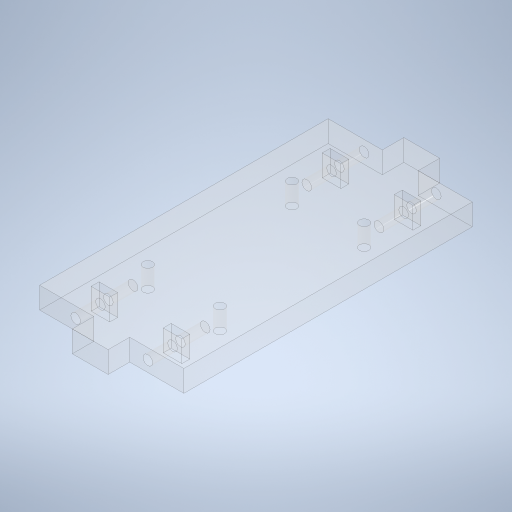
# Autodesk Inventor part: feet_holder3
Saved by Autodesk Inventor 2024 (Build 280153000, 153)
## iProperties
Created: 2024-09-07
Part Number: feet_holder3
Material: PMMA 플라스틱
Document SubType Name: Modeling
Designer: jmha0
Density: 1.188 g/cm^3
Appearance: 폴리카보네이트 - 선명
Mass: 23.3204 g
Surface Area: 87.9044 cm^2
Volume: 19.63 cm^3
Author: jmha0
Autodesk Inventor part; units mm, degrees
ref_plane "YZ Plane" through (0, 0, 0) normal (1, 0, 0) x (0, 1, 0)
ref_plane "XZ Plane" through (0, 0, 0) normal (0, 1, 0) x (-1, 0, 0)
ref_plane "XY Plane" through (0, 0, 0) normal (0, 0, 1) x (1, 0, 0)
sketch "스케치1" plane through (0, 0, 0) normal (0, 1, 0) x (-1, 0, 0)
  circle A0 centre (7.6948, -23.9851) radius 1.45
  circle A1 centre (27.7948, -23.9851) radius 1.45
  line L0 (-2.3552, -20.9851) -> (37.8448, -20.9851)
  line L1 (-2.3552, -20.9851) -> (-2.3552, -26.9851)
  line L2 (37.8448, -26.9851) -> (-2.3552, -26.9851)
  line L3 (37.8448, -20.9851) -> (37.8448, -26.9851)
  circle A2 centre (27.7948, 62.4149) radius 1.45
  circle A3 centre (7.6948, 62.4149) radius 1.45
  line L4 (37.8448, 65.4149) -> (-2.3552, 65.4149)
  line L5 (-2.3552, 65.4149) -> (-2.3552, 59.4149)
  line L6 (37.8448, 59.4149) -> (-2.3552, 59.4149)
  line L7 (37.8448, 65.4149) -> (37.8448, 59.4149)
  line L8 (37.8448, -20.9851) -> (-2.3552, -20.9851)
  line L9 (-2.3552, -20.9851) -> (-2.3552, 59.4149)
  line L10 (-2.3552, 59.4149) -> (37.8448, 59.4149)
  line L11 (37.8448, 59.4149) -> (37.8448, -20.9851)
  point P0 (0, 0)
  constraints: 24 end point, 4 centre point, 2 parallel, 1 horizontal, 1 perpendicular
extrude "돌출1" add sketch "스케치1" along normal blind 6 contours L9 L6 L11 L0
sketch "스케치2" plane through (0, 6, 0) normal (0, 1, 0) x (1, 0, 0)
  line L0 (2.3552, 20.9851) -> (-37.8448, 20.9851) projected
  line L1 (-37.8448, 20.9851) -> (-37.8448, -59.4149) projected
  line L2 (-37.8448, -59.4149) -> (2.3552, -59.4149) projected
  line L3 (2.3552, -59.4149) -> (2.3552, 20.9851) projected
  line L4 (-47.7448, 30.7851) -> (12.2552, -69.2149) construction
  line L5 (12.2552, 30.7851) -> (-47.7448, -69.2149) construction
  circle A0 centre (-7.6948, -39.3149) radius 1.35
  circle A1 centre (-27.7948, -39.3149) radius 1.35
  circle A2 centre (-7.6948, 0.8851) radius 1.35
  circle A3 centre (-27.7948, 0.8851) radius 1.35
  point P0 (0, 0)
  dimension "d2" = 60
  dimension "d3" = 100
  dimension "d4" = 2.7
  dimension "d5" = 2.7
  dimension "d6" = 2.7
  dimension "d27" = 2.7
  constraints: 4 centre point, 4 end point
  measures "d2" distance of L4.end L5.end
  measures "d3" distance of L5.start L4.end
  measures "d4" diameter of A0
  measures "d5" diameter of A2
  measures "d6" diameter of A3
  measures "d27" diameter of A1
extrude "돌출2" cut sketch "스케치2" against normal blind 6 contours A0 | A1 | A2 | A3
sketch "스케치3" plane through (-37.8448, 0, 59.4149) normal (0, 0, 1) x (1, 0, 0)
  line L0 (0, 0) -> (40.2, 0) projected
  line L1 (40.2, 0) -> (40.2, 6) projected
  line L2 (0, 6) -> (40.2, 6) projected
  line L3 (0, 0) -> (0, 6) projected
  line L4 (0, 6) -> (10.05, 6)
  line L5 (10.05, 6) -> (30.15, 6)
  circle A0 centre (10.05, 3) radius 1.35
  circle A1 centre (30.15, 3) radius 1.35
  point P0 (37.8448, 0)
  dimension "d9" = 40.2
  dimension "d10" = 6
  dimension "d11" = 10.05
  dimension "d12" = 20.1
  dimension "d13" = 2.7
  dimension "d14" = 2.7
  constraints: 4 end point, 2 centre point, 2 point on line
  measures "d9" distance of L2.start L1.end
  measures "d10" distance of L0.start L2.start
  measures "d11" distance of L2.start L4.end
  measures "d12" distance of L4.end L5.end
  measures "d13" diameter of A0
  measures "d14" diameter of A1
extrude "돌출3" cut sketch "스케치3" against normal blind 16 contours A0 | A1
sketch "스케치4" plane through (2.3552, 0, -20.9851) normal (0, 0, -1) x (-1, 0, 0)
  circle A0 centre (30.15, 3) radius 1.35 projected
  line L0 (11.4, 6) -> (11.4, 0) projected
  circle A1 centre (10.05, 3) radius 1.35 projected
  point P0 (2.3552, 0)
extrude "돌출4" cut sketch "스케치4" against normal blind 16
sketch "스케치5" plane through (0, 6, 0) normal (0, 1, 0) x (1, 0, 0)
  line L0 (-29.1448, 20.9851) -> (-29.1448, 4.9851) projected
  line L1 (-26.4448, 20.9851) -> (-26.4448, 4.9851) projected
  line L2 (-29.1448, 4.9851) -> (-26.4448, 4.9851) projected
  line L3 (-9.0448, 20.9851) -> (-9.0448, 4.9851) projected
  line L4 (-6.3448, 20.9851) -> (-6.3448, 4.9851) projected
  line L5 (-9.0448, 4.9851) -> (-6.3448, 4.9851) projected
  circle A0 centre (-7.6948, 0.8851) radius 1.35 projected
  circle A1 centre (-27.7948, 0.8851) radius 1.35 projected
  circle A2 centre (-7.6948, -39.3149) radius 1.35 projected
  circle A3 centre (-27.7948, -39.3149) radius 1.35 projected
  line L6 (2.3552, 20.9851) -> (-37.8448, 20.9851) projected
  line L7 (-37.8448, 20.9851) -> (-37.8448, -59.4149) projected
  line L8 (-37.8448, -59.4149) -> (2.3552, -59.4149) projected
  line L9 (2.3552, -59.4149) -> (2.3552, 20.9851) projected
  line L10 (-9.0448, -59.4149) -> (-9.0448, -43.4149) projected
  line L11 (-29.1448, -59.4149) -> (-29.1448, -43.4149) projected
  line L12 (-26.4448, -59.4149) -> (-26.4448, -43.4149) projected
  line L13 (-6.3448, -59.4149) -> (-6.3448, -43.4149) projected
  line L14 (-30.3948, -52.5149) -> (-25.1948, -52.5149)
  line L15 (-25.1948, -52.5149) -> (-25.1948, -50.3149)
  line L16 (-25.1948, -50.3149) -> (-30.3948, -50.3149)
  line L17 (-30.3948, -50.3149) -> (-30.3948, -52.5149)
  line L18 (-30.3948, -52.5149) -> (-25.1948, -50.3149) construction
  line L19 (-25.1948, -52.5149) -> (-30.3948, -50.3149) construction
  line L20 (-10.2948, -52.5149) -> (-5.0948, -52.5149)
  line L21 (-5.0948, -52.5149) -> (-5.0948, -50.3149)
  line L22 (-5.0948, -50.3149) -> (-10.2948, -50.3149)
  line L23 (-10.2948, -50.3149) -> (-10.2948, -52.5149)
  line L24 (-10.2948, -52.5149) -> (-5.0948, -50.3149) construction
  line L25 (-5.0948, -52.5149) -> (-10.2948, -50.3149) construction
  line L26 (-30.3948, 11.8851) -> (-25.1948, 11.8851)
  line L27 (-25.1948, 11.8851) -> (-25.1948, 14.0851)
  line L28 (-25.1948, 14.0851) -> (-30.3948, 14.0851)
  line L29 (-30.3948, 14.0851) -> (-30.3948, 11.8851)
  line L30 (-30.3948, 11.8851) -> (-25.1948, 14.0851) construction
  line L31 (-25.1948, 11.8851) -> (-30.3948, 14.0851) construction
  line L32 (-10.2948, 11.8851) -> (-5.0948, 11.8851)
  line L33 (-5.0948, 11.8851) -> (-5.0948, 14.0851)
  line L34 (-5.0948, 14.0851) -> (-10.2948, 14.0851)
  line L35 (-10.2948, 14.0851) -> (-10.2948, 11.8851)
  line L36 (-10.2948, 11.8851) -> (-5.0948, 14.0851) construction
  line L37 (-5.0948, 11.8851) -> (-10.2948, 14.0851) construction
  point P0 (0, 0)
  point P1 (-27.7948, -51.4149)
  point P2 (-7.6948, -51.4149)
  point P3 (-27.7948, 12.9851)
  point P4 (-7.6948, 12.9851)
  dimension "d34" = 5.2
  dimension "d35" = 2.2
  dimension "d36" = 5.2
  dimension "d37" = 2.2
  dimension "d38" = 5.2
  dimension "d39" = 2.2
  dimension "d40" = 5.2
  dimension "d41" = 2.2
  constraints: 48 end point, 8 midpoint, 8 parallel, 4 horizontal, 4 perpendicular
  measures "d34" distance of L16.end L15.end
  measures "d35" distance of L15.end L14.end
  measures "d36" distance of L22.end L21.end
  measures "d37" distance of L21.end L20.end
  measures "d38" distance of L28.end L27.end
  measures "d39" distance of L27.end L26.end
  measures "d40" distance of L34.end L33.end
  measures "d41" distance of L33.end L32.end
extrude "돌출5" cut sketch "스케치5" against normal blind 6 contours L28 L1 L26 L0 | L0 L26 L29 L28 | L28 L27 L26 L1 | L34 L4 L32 L3 | L3 L32 L35 L34 | L34 L33 L32 L4 | L14 L17 L16 L11 | L11 L16 L12 L14 | L12 L16 L15 L14 | L20 L23 L22 L10 | L10 L22 L13 L20 | L13 L22 L21 L20
sketch "스케치6" plane through (-37.8448, 0, 59.4149) normal (0, 0, 1) x (1, 0, 0)
  circle A0 centre (30.15, 3) radius 1.35 projected
  circle A1 centre (10.05, 3) radius 1.35 projected
  line L0 (0, 0) -> (40.2, 0) projected
  line L1 (40.2, 0) -> (40.2, 6) projected
  line L2 (0, 6) -> (40.2, 6) projected
  line L3 (0, 0) -> (0, 6) projected
  line L4 (15.1, 0) -> (25.1, 0)
  line L5 (25.1, 0) -> (25.1, 6)
  line L6 (25.1, 6) -> (15.1, 6)
  line L7 (15.1, 6) -> (15.1, 0)
  line L8 (15.1, 0) -> (25.1, 6) construction
  line L9 (25.1, 0) -> (15.1, 6) construction
  point P0 (37.8448, 0)
  point P1 (20.1, 3)
  dimension "d28" = 10
  constraints: 12 end point, 2 midpoint, 2 parallel, 1 horizontal, 1 perpendicular, 1 point on line
  measures "d28" distance of L6.end L5.end
extrude "돌출6" add sketch "스케치6" along normal blind 6 contours L7 L2 L5 L0
sketch "스케치7" plane through (2.3552, 0, -20.9851) normal (0, 0, -1) x (-1, 0, 0)
  line L0 (15.1, 6) -> (15.1, 0) projected
  line L1 (25.1, 0) -> (25.1, 6) projected
  circle A0 centre (30.15, 3) radius 1.35 projected
  circle A1 centre (10.05, 3) radius 1.35 projected
  line L2 (0, 0) -> (40.2, 0) projected
  line L3 (40.2, 0) -> (40.2, 6) projected
  line L4 (0, 6) -> (40.2, 6) projected
  line L5 (0, 0) -> (0, 6) projected
  point P0 (2.3552, 0)
extrude "돌출7" add sketch "스케치7" along normal blind 6 contours L4 L1 L2 L0
